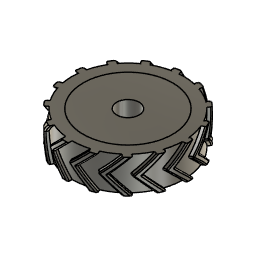
llanta (Autodesk Fusion 360 design; units mm, degrees)
Autodesk Fusion 360 part; units mm, degrees
note: some values were not read from the file. Chosen so that the rebuilt part matches the saved one: where a step starts.
sketch "Boceto1" plane through (0, 0, 0) normal (0, 0, 1) x (1, 0, 0)
  circle A0 centre (0, 0) radius 50
  circle A1 centre (0, 0) radius 40
  dimension "d1" = 100
  dimension "d2" = -10
  constraint coincident A0.centre A1.centre
  measures "d1" diameter of A0
extrude "Extruir1" add sketch "Boceto1" along normal blind 30 makes body 1
sketch "Boceto2" plane through (0, 0, 0) normal (0, 1, 0) x (1, 0, 0)
  line L0 (-50, -30) -> (50, -30)
  line L1 (-50, 0) -> (50, 0)
  line L2 (0, 0) -> (0, -30) construction
  line L3 (0, -15) -> (-15, -15) construction
  line L4 (0, 0) -> (-15, -15)
  line L5 (-15, -15) -> (0, -30)
  line L6 (-6.364, 0) -> (-21.364, -15)
  line L7 (-21.364, -15) -> (-6.364, -30)
  dimension "d5" = 15
  constraint coincident L2.start L4.start
  constraint midpoint L0 L2.end
  constraint midpoint L2 L3.start
  constraint perpendicular L2 L3
  constraint coincident L1 L6.start
  constraint coincident L0 L7.end
  measures "d5" distance of L3.start L3.end
extrude "Extruir2" add sketch "Boceto2" against normal blind 3.5 from the far side of the face at (49.7515, -4.9784, 20) on bodies 1 bodies 1
fillet "Empalme1" radius 1 5 edges at (-21.364, -46.956, 15) (-14.0364, -51.4894, 22.3275) (-14.0364, -51.4894, 7.6725) (-7.5879, -52.9209, 22.4121) (-7.5879, -52.9209, 7.5879) on bodies 1
pattern_circular "Patrón C1" count 15 over 360 about axis through (0, 0, 0) along (0, 0, 1) of "Extruir2", "Empalme1"
extrude "Extruir3" add sketch "Boceto1" along normal blind 30 separate body contours A1 makes body 2
sketch "Boceto3" plane through (0, 0, 30) normal (0, 0, 1) x (-1, 0, 0)
  circle A0 centre (0, 0) radius 40
  circle A1 centre (0, 0) radius 10
  dimension "d15" = 20
  constraint concentric A0 A1
  measures "d15" diameter of A1
extrude "Extruir4" cut sketch "Boceto3" against normal through all contours A1 bodies 2
named bodies: "Llanta", "Rin"
